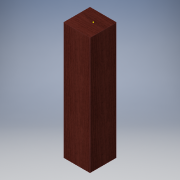
# Autodesk Inventor part: stand
Saved by Autodesk Inventor 2019 (Build 230136000, 136)
## iProperties
Created: 2019-04-29
Part Number: stand
Material: Wood (Birch)
Document SubType Name: Modeling
Designer: Alex
Density: 0.55 g/cm^3
Appearance: Birch - Natural Polished
Author: Alex
Autodesk Inventor part; units mm, degrees
ref_plane "YZ Plane" through (0, 0, 0) normal (1, 0, 0) x (0, 1, 0)
ref_plane "XZ Plane" through (0, 0, 0) normal (0, 1, 0) x (-1, 0, 0)
ref_plane "XY Plane" through (0, 0, 0) normal (0, 0, 1) x (1, 0, 0)
sketch "Sketch1" plane through (0, 0, 0) normal (0, 1, 0) x (-1, 0, 0)
  line L0 (83.1496, 85.748) -> (-66.8504, 85.748)
  line L1 (-66.8504, 85.748) -> (-66.8504, -64.252)
  line L2 (-66.8504, -64.252) -> (83.1496, -64.252)
  line L3 (83.1496, -64.252) -> (83.1496, 85.748)
  point P0 (0, 0)
  dimension "d1" = 150
  dimension "d4" = 150
  constraints: 8 end point, 2 parallel, 1 horizontal, 1 perpendicular
  measures "d1" distance between parallel lines of L1 L3
  measures "d4" distance between parallel lines of L2 L0
extrude "Extrusion1" add sketch "Sketch1" along normal blind 660
sketch "Sketch2" plane through (0, 660, 0) normal (0, 1, 0) x (1, 0, 0)
  point P0 (0, 0)
sketch "Sketch3" plane through (0, 660, 0) normal (0, 1, 0) x (1, 0, 0)
  point P0 (0, 0)
sketch "Sketch4" plane through (0, 660, 0) normal (0, 1, 0) x (1, 0, 0)
  point P0 (0, 0)
fillet "Fillet1" radius 3 4 edges at (66.8504, 330, 85.748) (-83.1496, 330, 85.748) (66.8504, 330, -64.252) (-83.1496, 330, -64.252)
body "Solid1"
